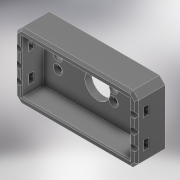
# Autodesk Inventor part: 4
Saved by Autodesk Inventor 2022 (Build 260153000, 153)
## iProperties
Company: HS Emden/Leer
Created: 2023-12-24
Part Number: 4
Material: PMMA-Kunststoff
Document SubType Name: Modeling
Designer: Yaman Alsaady
Density: 1.188 g/cm^3
Appearance: Glatt - Schwarz
Project: Delta-Robot
Author: Yaman Alsaady
Title: Caver
## iProperties of the stored document 2_3D-Druck.ipt
Created: 2023-12-24
Part Number: 2_3D-Druck
Material: Generisch
Document SubType Name: Modeling
Designer: alsaa
Density: 1 g/cm^3
Appearance: Vorgabe
Author: alsaa
Autodesk Inventor part; units mm, degrees
ref_plane "YZ Plane" through (0, 0, 0) normal (1, 0, 0) x (0, 1, 0)
ref_plane "XZ Plane" through (0, 0, 0) normal (0, 1, 0) x (-1, 0, 0)
ref_plane "XY Plane" through (0, 0, 0) normal (0, 0, 1) x (1, 0, 0)
sketch "Skizze1" plane through (0, 0, 0) normal (0, 0, 1) x (1, 0, 0)
  line L0 (47, -23) -> (-47, -23)
  line L1 (-47, -23) -> (-47, 23)
  line L2 (-47, 23) -> (47, 23)
  line L3 (47, 23) -> (47, -23)
  line L4 (47, -23) -> (-47, 23) construction
  line L5 (-47, -23) -> (47, 23) construction
  circle A0 centre (0, 0) radius 11
  dimension "d1" = 46
  dimension "d8" = 22
  dimension "d9" = 47
  constraints: 12 end point, 2 midpoint, 2 parallel, 1 centre point, 1 coincident, 1 horizontal, 1 perpendicular
  measures "d1" distance of L2.end L0.start
  measures "d8" diameter of A0
  measures "d9" distance from line of L3 point (0, 0)
extrude "Extrusion1" add sketch "Skizze1" along normal blind 6
sketch "Skizze2" plane through (0, 0, 6) normal (0, 0, 1) x (1, 0, 0)
  line L0 (53, -29) -> (-53, -29)
  line L1 (-53, -29) -> (-53, 29)
  line L2 (-53, 29) -> (53, 29)
  line L3 (53, 29) -> (53, -29)
  line L4 (53, -29) -> (-53, 29) construction
  line L5 (-53, -29) -> (53, 29) construction
  line L6 (47, 23) -> (-47, 23) projected
  line L7 (-47, 23) -> (-47, -23) projected
  line L8 (-47, -23) -> (47, -23) projected
  line L9 (47, -23) -> (47, 23) projected
  point P0 (0, 0)
  dimension "d10" = 6
  dimension "d11" = 6
  constraints: 12 end point, 2 midpoint, 2 parallel, 1 horizontal, 1 perpendicular
  measures "d10" distance between parallel lines of L3 L9
  measures "d11" distance between parallel lines of L6 L2
extrude "Extrusion2" add sketch "Skizze2" along normal blind 19 and the other way blind 6
sketch "Skizze3" plane through (-53, -29, 25) normal (-1, 0, 0) x (0, 0, 1)
  line L0 (-19, 52) -> (-19, 6) projected
  line L1 (-19, 52) -> (0, 52) projected
  line L2 (0, 6) -> (0, 52) projected
  line L3 (-19, 6) -> (0, 6) projected
  line L4 (-12, 19) -> (-19, 19)
  line L5 (-19, 19) -> (-19, 39)
  line L6 (-19, 39) -> (-12, 39)
  line L7 (-12, 39) -> (-12, 19)
  line L8 (0, 52) -> (-19, 52) projected
  line L9 (-12, 52) -> (-12, 6)
  point P0 (-25, 29)
  point P1 (-19, 29)
  point P2 (-19, 39)
  point P3 (-19, 19)
  point P4 (-12, 29)
  point P5 (-12, 39)
  point P6 (-12, 52)
  point P7 (-12, 19)
  dimension "d14" = 20
  dimension "d15" = 7
  constraints: 10 end point, 4 midpoint, 2 parallel, 2 perpendicular, 2 point on line, 1 horizontal
  measures "d14" distance between parallel lines of L4 L6
  measures "d15" distance of L4.start L4.end
extrude "Extrusion3" [suppressed]
extrude "Extrusion4" [suppressed]
sketch "Skizze5" plane through (0, 0, 25) normal (0, 0, 1) x (1, 0, 0)
  line L0 (53, 29) -> (53, -29) construction
  line L1 (53, 0) -> (47, 0) construction
  line L2 (47, -23) -> (47, 23) construction
  line L3 (47, 23) -> (-47, 23) construction
  line L4 (0, 23) -> (0, -23) construction
  circle A0 centre (50, 0) radius 1.85
  circle A1 centre (-50, 0) radius 1.85
  point P0 (0, 0)
  point P1 (0, 0)
  dimension "d23" = 3.7
  constraints: 5 midpoint, 4 end point, 2 centre point, 1 coincident, 1 symmetric about line, 1 other
  measures "d23" diameter of A0
extrude "Extrusion5" cut sketch "Skizze5" against normal through all
sketch "Skizze6" plane through (0, 0, 0) normal (0, 0, -1) x (-1, 0, 0)
  circle A0 centre (-50, 0) radius 1.85 projected
  line L0 (-50, -3.4641) -> (-53, -1.7321)
  line L1 (-53, -1.7321) -> (-53, 1.7321)
  line L2 (-53, 1.7321) -> (-50, 3.4641)
  line L3 (-50, 3.4641) -> (-47, 1.7321)
  line L4 (-47, 1.7321) -> (-47, -1.7321)
  line L5 (-47, -1.7321) -> (-50, -3.4641)
  line L6 (-53, 29) -> (-53, -29) projected
  line L7 (-53, -29) -> (53, -29) construction
  line L8 (0, -29) -> (0, 29) construction
  line L9 (53, 29) -> (-53, 29) construction
  circle A1 centre (50, 0) radius 1.85
  line L10 (50, -3.4641) -> (53, -1.7321)
  line L11 (53, -1.7321) -> (53, 1.7321)
  line L12 (53, 1.7321) -> (50, 3.4641)
  line L13 (50, 3.4641) -> (47, 1.7321)
  line L14 (47, 1.7321) -> (47, -1.7321)
  line L15 (47, -1.7321) -> (50, -3.4641)
  point P0 (0, 0)
  dimension "d26" = 6
  constraints: 26 end point, 7 symmetric about line, 2 midpoint, 1 centre point, 1 coincident, 1 collinear, 14 other
  measures "d26" distance between parallel lines of L4 L1
extrude "Extrusion6" cut sketch "Skizze6" against normal blind 3 contours A0 | L0 L1 L2 L3 L4 L5 | L15 L14 L13 L12 L11 L10
sketch "Skizze7" plane through (0, 0, 0) normal (0, 0, -1) x (-1, 0, 0)
  line L0 (-53, -29) -> (53, -29) construction
  line L1 (10.25, -29) -> (10.25, 29) construction
  line L2 (53, 29) -> (-53, 29) construction
  line L3 (53, 0) -> (-52.7245, 0) construction
  circle A0 centre (-14, -5) radius 2.15
  circle A1 centre (-14, 5) radius 2.15
  circle A2 centre (34.5, 5) radius 2.15
  circle A3 centre (34.5, -5) radius 2.15
  line L4 (53, -29) -> (53, 29) projected
  point P0 (0, 0)
  dimension "d29" = 10.25
  dimension "d30" = 48.5
  dimension "d31" = 10
  dimension "d32" = 4.3
  constraints: 4 centre point, 4 end point, 3 equal radius, 3 symmetric about line, 2 point on line, 1 horizontal, 1 midpoint, 1 vertical
  measures "d29" distance from line of point (0, 0) L1
  measures "d30" distance of A1.centre A2.centre
  measures "d31" distance of A0.centre A1.centre
  measures "d32" diameter of A3
extrude "Extrusion7" cut sketch "Skizze7" against normal through all
fillet "Rundung1" radius 2 4 edges at (-32.35, -5, 6) (-32.35, 5, 6) (16.15, 5, 6) (16.15, -5, 6)
chamfer "Fase1" distance 5 angle 45 4 edges at (-53, -29, 12.5) (53, -29, 12.5) (53, 29, 12.5) (-53, 29, 12.5)
chamfer "Fase2" [suppressed]
fillet "Rundung2" [suppressed]
chamfer "Fase3" [suppressed]
sketch "Skizze8" plane through (0, 0, 6) normal (0, 0, 1) x (1, 0, 0)
  circle A0 centre (-50, 17.5) radius 1.65 projected
  line L0 (-53, 19.5791) -> (-53, 15.4209) projected
  arc A1 (-53, 15.4209) -> (-53, 19.5791) centre (-50, 17.5) ccw projected
  circle A2 centre (50, 17.5) radius 1.65 projected
  line L1 (53, 15.4209) -> (53, 19.5791) projected
  arc A3 (53, 19.5791) -> (53, 15.4209) centre (50, 17.5) ccw projected
extrude "Extrusion8" [suppressed]
sketch "Skizze9" plane through (53, -1.7321, 3) normal (1, 0, 0) x (0, 0, -1)
  line L0 (3, 1.7321) -> (-22, 1.7321) construction
  line L1 (-22, -22.2679) -> (-22, 25.7321) construction
  line L2 (-15.8, 10.0821) -> (-11.5, 10.0821)
  line L3 (-11.5, 10.0821) -> (-11.5, 18.3821)
  line L4 (-11.5, 18.3821) -> (-15.8, 18.3821)
  line L5 (-15.8, 18.3821) -> (-15.8, 10.0821)
  line L6 (-3, 24.7321) -> (-3, -21.2679) projected
  line L7 (-3, -21.2679) -> (-3, 24.7321) projected
  line L8 (-3, -7.4179) -> (-3, 0.8821) projected
  line L9 (-3, 0.8821) -> (-3, -7.4179) projected
  line L10 (-3, -3.1619) -> (-3, -0.7219) projected
  line L11 (-3, -3.1619) -> (-3, 6.626) projected
  line L12 (-3, 4.186) -> (-3, 6.626) projected
  line L13 (-15.8, -6.6179) -> (-11.5, -6.6179)
  line L14 (-11.5, -6.6179) -> (-11.5, -14.9179)
  line L15 (-11.5, -14.9179) -> (-15.8, -14.9179)
  line L16 (-15.8, -14.9179) -> (-15.8, -6.6179)
  line L17 (-3, 4.186) -> (-3, -0.7219) projected
  point P0 (-11.5, -10.7679)
  point P1 (-11.5, 14.2321)
  dimension "d49" = 4.3
  dimension "d50" = 8.5
  dimension "d54" = 25
  dimension "d55" = 8.3
  constraints: 18 end point, 4 symmetric about line, 3 midpoint, 2 parallel, 1 horizontal, 1 perpendicular
  measures "d49" distance of L2.start L2.end
  measures "d50" distance between parallel lines of L6 L3
  measures "d54" distance of point (-11.5, 14.232) point (-11.5, -10.768)
  measures "d55" distance of L4.end L2.start
extrude "Extrusion9" cut sketch "Skizze9" against normal through all
sketch "Skizze10" plane through (0, 0, 3) normal (0, 0, -1) x (-1, 0, 0)
  circle A0 centre (-50, 0) radius 1.85 projected
  line L0 (-47, 1.7321) -> (-47, -1.7321) projected
  line L1 (-50, 3.4641) -> (-47, 1.7321) projected
  line L2 (-53, 1.7321) -> (-50, 3.4641) projected
  line L3 (-53, -1.7321) -> (-53, 1.7321) projected
  line L4 (-50, -3.4641) -> (-53, -1.7321) projected
  line L5 (-47, -1.7321) -> (-50, -3.4641) projected
  circle A1 centre (50, 0) radius 1.85 projected
  line L6 (53, 1.7321) -> (53, -1.7321) projected
  line L7 (50, 3.4641) -> (53, 1.7321) projected
  line L8 (47, 1.7321) -> (50, 3.4641) projected
  line L9 (47, -1.7321) -> (47, 1.7321) projected
  line L10 (50, -3.4641) -> (47, -1.7321) projected
  line L11 (53, -1.7321) -> (50, -3.4641) projected
  point P0 (0, 0)
extrude "Extrusion10" add sketch "Skizze10" along normal up to surface (3 mm away)
sketch "Skizze11" plane through (0, 0, 25) normal (0, 0, 1) x (1, 0, 0)
  line L0 (-50, 12.5) -> (-50, -12.5) construction
  circle A0 centre (-50, 0) radius 1.85 construction
  circle A1 centre (50, 0) radius 1.85 construction
  line L1 (50, 12.5) -> (50, -12.5) construction
  circle A2 centre (-50, 12.5) radius 1.85
  circle A3 centre (-50, -12.5) radius 1.85
  line L2 (-47, 23) -> (-47, -23) projected
  circle A4 centre (50, 12.5) radius 1.85
  circle A5 centre (50, -12.5) radius 1.85
  point P0 (0, 0)
  dimension "d59" = 25
  constraints: 6 coincident, 4 centre point, 4 end point, 4 equal radius, 2 midpoint, 2 vertical, 1 parallel
  measures "d59" distance of L1.start L1.end
extrude "Extrusion11" cut sketch "Skizze11" against normal through all
chamfer "Fase4" distance 2 angle 45 8 edges at (0, 29, 25) (-50.5, 26.5, 25) (-53, 0, 25) (-50.5, -26.5, 25) (0, -29, 25) (50.5, -26.5, 25) (53, 0, 25) (50.5, 26.5, 25)
chamfer "Fase5" distance 1 angle 45 4 edges at (-47, 0, 25) (0, 23, 25) (47, 0, 25) (0, -23, 25)
sketch "Skizze12" plane through (0, 0, 25) normal (0, 0, 1) x (1, 0, 0)
  circle A0 centre (-50, 12.5) radius 1.85 projected
  circle A1 centre (-50, 0) radius 1.85 projected
  circle A2 centre (-50, -12.5) radius 1.85 projected
  circle A3 centre (50, 12.5) radius 1.85 projected
  circle A4 centre (50, 0) radius 1.85 projected
  circle A5 centre (50, -12.5) radius 1.85 projected
  circle A6 centre (-50, 12.5) radius 2.75
  circle A7 centre (-50, 0) radius 2.75
  circle A8 centre (-50, -12.5) radius 2.75
  circle A9 centre (50, 12.5) radius 1.85 projected
  circle A10 centre (50, 12.5) radius 2.75
  circle A11 centre (50, 0) radius 2.75
  circle A12 centre (50, -12.5) radius 1.85 projected
  circle A13 centre (50, -12.5) radius 2.75
  point P0 (0, 0)
  dimension "d68" = 5.5
  constraints: 6 centre point, 6 coincident, 5 equal radius
  measures "d68" diameter of A6
extrude "Extrusion12" cut sketch "Skizze12" against normal blind 4 contours A0 | A1 | A2 | A3 | A6 | A7 | A8 | A10 | A11 | A13
equation "\"d11\" = d10"
